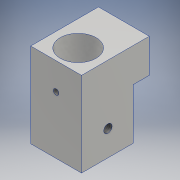
# Autodesk Inventor part: carro_do_rolamento_direito
Saved by Autodesk Inventor 2018 (Build 220112000, 112)
## iProperties
Created: 2018-05-16
Part Number: carro_do_rolamento_direito
Material: Alumínio 6061
Document SubType Name: Modeling
Designer: Usuario
Density: 2.7 g/cm^3
Appearance: Alumínio - Plano
Author: Usuario
Autodesk Inventor part; units mm, degrees
ref_plane "YZ Plane" through (0, 0, 0) normal (1, 0, 0) x (0, 1, 0)
ref_plane "XZ Plane" through (0, 0, 0) normal (0, 1, 0) x (-1, 0, 0)
ref_plane "XY Plane" through (0, 0, 0) normal (0, 0, 1) x (1, 0, 0)
sketch "Esboço1" plane through (0, 0, 0) normal (0, 0, 1) x (1, 0, 0)
  circle A0 centre (9.5, -2.575) radius 10.5 construction
  line L0 (21.9348, 5.0533) -> (21.9348, -29.9467) construction
  line L1 (-3.0652, -29.9467) -> (-3.0652, 5.0533) construction
  circle A1 centre (9.5, -2.575) radius 10.575 construction
  line L2 (21.9348, -13.15) -> (-3.0652, -13.15) construction
  line L3 (9.4348, -13.15) -> (9.4348, 4.425) construction
  line L4 (-5.5652, 24.425) -> (24.4348, 24.425)
  line L5 (24.4348, 24.425) -> (24.4348, -15.575)
  line L6 (24.4348, -15.575) -> (-5.5652, -15.575)
  line L7 (-5.5652, -15.575) -> (-5.5652, 24.425)
  line L8 (-5.5652, 24.425) -> (24.4348, -15.575) construction
  line L9 (24.4348, 24.425) -> (-5.5652, -15.575) construction
  point P0 (0, 0)
  dimension "d1" = 21.15
  dimension "d3" = 30
  dimension "d4" = 40
  dimension "d51" = 13
  constraints: 20 end point, 3 midpoint, 2 centre point, 2 horizontal, 2 parallel, 2 perpendicular, 2 point on line, 1 coincident, 1 tangent
  measures "d1" diameter of A1
  measures "d3" distance of L5.end L6.end
  measures "d4" distance of L4.end L5.end
  measures "d51" distance from line of L6 A0.centre
extrude "Extrusão1" add sketch "Esboço1" against normal blind 50
sketch "Esboço2" plane through (0, 0, 0) normal (0, 0, 1) x (1, 0, 0)
  circle A0 centre (9.4348, -2.575) radius 5.995 construction
  line L0 (24.4348, -15.575) -> (-5.5652, -15.575) projected
  line L1 (-5.5652, -15.575) -> (-5.5652, 24.425) projected
  dimension "d52" = 13
  dimension "d53" = 15
  constraints: 1 centre point
  measures "d52" distance from line of L0 A0.centre
  measures "d53" distance from line of L1 A0.centre
hole "Furo1" at (9.4348, -2.575, 0) direction (0, 0, -1) diameter 13 end through all counterbore diameter 21.2 counterbore depth 32
sketch "Esboço3" plane through (-5.5652, -15.575, 0) normal (-1, 0, 0) x (0, 0, 1)
  line L0 (-50, 0) -> (-50, 40) construction
  line L1 (0, 40) -> (0, 0) construction
  line L2 (-50, 40) -> (0, 40) construction
  line L3 (0, 40) -> (0, 0) construction
  line L4 (0, 0) -> (-50, 0) construction
  line L5 (-50, 0) -> (-50, 40) construction
  line L6 (0, 15.575) -> (-50, 15.575) construction
  line L7 (-35, 15.575) -> (-35, 40) construction
  constraints: 12 end point, 3 perpendicular, 3 point on line, 2 parallel, 1 horizontal
hole "Furo2" at (-5.5652, 0, -35) direction (1, 0, 0) diameter 4.917 depth 13 tip angle 118 thread size "M6x1" class "6H" standard "ANSI Metric M Profile"
sketch "Esboço4" plane through (-5.5652, -15.575, 0) normal (-1, 0, 0) x (0, 0, 1)
  line L0 (-50, 30.5) -> (-20, 30.5)
  line L1 (-20, 30.5) -> (-20, 40)
  line L2 (-20, 40) -> (-50, 40)
  line L3 (-50, 40) -> (-50, 30.5)
  point P0 (0, 15.575)
  point P1 (-50, 0)
  dimension "d22" = 30.5
  dimension "d23" = 30
  constraints: 8 end point, 2 perpendicular
  measures "d22" distance of point (-50, 0) L0.start
  measures "d23" distance of L0.start L0.end
extrude "Extrusão2" cut sketch "Esboço4" against normal blind 31.25
sketch "Esboço6" plane through (24.4348, -15.575, 0) normal (1, 0, 0) x (0, 0, -1)
  circle A0 centre (35, 15.575) radius 2.4585 construction
  circle A1 centre (35, 15.575) radius 2.4585 construction
  point P0 (0, 15.575)
  constraints: 1 centre point, 1 coincident
hole "Furo3" at (24.4348, 0, -35) direction (-1, 0, 0) diameter 4.917 depth 13 tip angle 118 thread size "M6x1" class "6H" standard "ANSI Metric M Profile"
sketch "Esboço7" plane through (-5.5652, -15.575, 0) normal (0, -1, 0) x (1, 0, 0)
  line L0 (0, 0) -> (30, 0) projected
  line L1 (15, 0) -> (15, -16) construction
  point P0 (5.5652, 0)
  dimension "d33" = 16
  constraints: 2 end point, 1 midpoint, 1 vertical
  measures "d33" distance of L1.start L1.end
hole "Furo4" at (9.4348, -15.575, -16) direction (0, 1, 0) diameter 3.242 depth 5.18 tip angle 118 thread size "M4x0.7" class "6H" standard "ANSI Metric M Profile"
sketch "Esboço8" plane through (-5.5652, 14.925, -20) normal (0, 1, 0) x (1, 0, 0)
  line L0 (30, 0) -> (0, 0) projected
  line L1 (30, 30) -> (0, 30) projected
  line L2 (30, -20) -> (30, 30) projected
  line L3 (0, -20) -> (0, 30) projected
  line L4 (15, 0) -> (15, 7.5) construction
  line L5 (15, 30) -> (15, 22.5) construction
  point P0 (5.5652, -20)
  dimension "d41" = 7.5
  dimension "d42" = 7.5
  constraints: 4 end point, 2 midpoint, 2 vertical
  measures "d41" distance of L4.start L4.end
  measures "d42" distance of L5.start L5.end
hole "Furo5" at (9.4348, 14.925, -27.5) at (9.4348, 14.925, -42.5) direction (0, -1, 0) diameter 3.242 depth 5.5 tip angle 118 thread size "M4x0.7" class "6H" standard "ANSI Metric M Profile"
